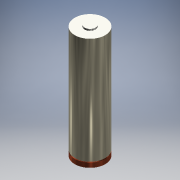
# Autodesk Inventor part: 18650
Saved by Autodesk Inventor 2017 (Build 210142000, 142)
## iProperties
Part Number: 18650
Material: Nickel-Kupfer-Legierung 400
Document SubType Name: Modeling
Designer: David Merges
Density: 8.83 g/cm^3
Appearance: Nickel
Author: David Merges
Autodesk Inventor part; units mm, degrees
ref_plane "YZ Plane" through (0, 0, 0) normal (1, 0, 0) x (0, 1, 0)
ref_plane "XZ Plane" through (0, 0, 0) normal (0, 1, 0) x (-1, 0, 0)
ref_plane "XY Plane" through (0, 0, 0) normal (0, 0, 1) x (1, 0, 0)
sketch "Skizze1" plane through (0, 0, 0) normal (0, 0, 1) x (1, 0, 0)
  circle A0 centre (0, 0) radius 9.25
  dimension "d0" = 18.5
  constraints: 1 centre point, 1 coincident
  measures "d0" diameter of A0
extrude "Extrusion1" add sketch "Skizze1" along normal mid plane 69
sketch "Skizze2" plane through (0, 0, 34.5) normal (0, 0, 1) x (1, 0, 0)
  circle A0 centre (0, 0) radius 3.3
  circle A1 centre (0, 0) radius 9.25 projected
  dimension "d3" = 6.6
  constraints: 1 centre point, 1 coincident
  measures "d3" diameter of A0
extrude "Extrusion2" cut sketch "Skizze2" against normal blind 1
sketch "Skizze3" plane through (0, 0, 0) normal (0, 1, 0) x (-1, 0, 0)
  line L0 (9.25, -34.5) -> (9.25, 33.5) construction
  line L1 (9.25, -31.25) -> (9, -31.5)
  line L2 (9, -31.5) -> (9.25, -31.75)
  line L3 (-9.25, -34.5) -> (9.25, -34.5) projected
  line L4 (9.25, -31.75) -> (9.25, -31.25)
  line L5 (0, -46.714) -> (0, 45.714) projected
  point P0 (0, 0)
  dimension "d6" = 3
  dimension "d7" = 0.5
  constraints: 6 end point, 2 perpendicular, 2 point on line, 1 collinear
  measures "d6" distance from line of L1.end L3
  measures "d7" distance of L2.end L1.start
revolve "Umdrehung1" cut sketch "Skizze3" angle 360 about axis through (0, 0, -10) along (0, 0, 1)
